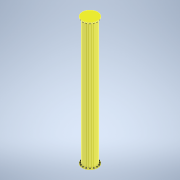
# Autodesk Inventor part: diam1m_len10m_x32gon_bolts
Saved by Autodesk Inventor 2022 (Build 260153000, 153)
## iProperties
Created: 2021-12-16
Part Number: diam1m_len10m_x32gon_bolts
Material: Steel
Document SubType Name: Modeling
Designer: jpc
Density: 7.85 g/cm^3
Appearance: Plate
Mass: 6.15675e+07 g
Surface Area: 349231 cm^2
Volume: 7.84299e+06 cm^3
Author: jpc
Autodesk Inventor part; units mm, degrees
ref_plane "YZ Plane" through (0, 0, 0) normal (1, 0, 0) x (0, 1, 0)
ref_plane "XZ Plane" through (0, 0, 0) normal (0, 1, 0) x (-1, 0, 0)
ref_plane "XY Plane" through (0, 0, 0) normal (0, 0, 1) x (1, 0, 0)
sketch "Sketch1" plane through (0, 0, 0) normal (0, 1, 0) x (-1, 0, 0)
  circle A0 centre (0, 0) radius 500 construction
  line L0 (497.5924, 49.0086) -> (497.5924, -49.0086)
  line L1 (497.5924, -49.0086) -> (478.4702, -145.1423)
  line L2 (478.4702, -145.1423) -> (440.9606, -235.6984)
  line L3 (440.9606, -235.6984) -> (386.5052, -317.1966)
  line L4 (386.5052, -317.1966) -> (317.1966, -386.5052)
  line L5 (317.1966, -386.5052) -> (235.6984, -440.9606)
  line L6 (235.6984, -440.9606) -> (145.1423, -478.4702)
  line L7 (145.1423, -478.4702) -> (49.0086, -497.5924)
  line L8 (49.0086, -497.5924) -> (-49.0086, -497.5924)
  line L9 (-49.0086, -497.5924) -> (-145.1423, -478.4702)
  line L10 (-145.1423, -478.4702) -> (-235.6984, -440.9606)
  line L11 (-235.6984, -440.9606) -> (-317.1966, -386.5052)
  line L12 (-317.1966, -386.5052) -> (-386.5052, -317.1966)
  line L13 (-386.5052, -317.1966) -> (-440.9606, -235.6984)
  line L14 (-440.9606, -235.6984) -> (-478.4702, -145.1423)
  line L15 (-478.4702, -145.1423) -> (-497.5924, -49.0086)
  line L16 (-497.5924, -49.0086) -> (-497.5924, 49.0086)
  line L17 (-497.5924, 49.0086) -> (-478.4702, 145.1423)
  line L18 (-478.4702, 145.1423) -> (-440.9606, 235.6984)
  line L19 (-440.9606, 235.6984) -> (-386.5052, 317.1966)
  line L20 (-386.5052, 317.1966) -> (-317.1966, 386.5052)
  line L21 (-317.1966, 386.5052) -> (-235.6984, 440.9606)
  line L22 (-235.6984, 440.9606) -> (-145.1423, 478.4702)
  line L23 (-145.1423, 478.4702) -> (-49.0086, 497.5924)
  line L24 (-49.0086, 497.5924) -> (49.0086, 497.5924)
  line L25 (49.0086, 497.5924) -> (145.1423, 478.4702)
  line L26 (145.1423, 478.4702) -> (235.6984, 440.9606)
  line L27 (235.6984, 440.9606) -> (317.1966, 386.5052)
  line L28 (317.1966, 386.5052) -> (386.5052, 317.1966)
  line L29 (386.5052, 317.1966) -> (440.9606, 235.6984)
  line L30 (440.9606, 235.6984) -> (478.4702, 145.1423)
  line L31 (478.4702, 145.1423) -> (497.5924, 49.0086)
  dimension "diamO" = 1000
  constraints: 64 end point, 2 coincident, 1 vertical, 68 other
extrude "Cylinder" add sketch "Sketch1" along normal blind 10000
sketch "Sketch2" plane through (0, 0, 0) normal (0, -1, 0) x (1, 0, 0)
  circle A0 centre (0, 0) radius 600 construction
  line L0 (597.1108, 58.8103) -> (597.1108, -58.8103)
  line L1 (597.1108, -58.8103) -> (574.1642, -174.1708)
  line L2 (574.1642, -174.1708) -> (529.1528, -282.838)
  line L3 (529.1528, -282.838) -> (463.8063, -380.636)
  line L4 (463.8063, -380.636) -> (380.636, -463.8063)
  line L5 (380.636, -463.8063) -> (282.838, -529.1528)
  line L6 (282.838, -529.1528) -> (174.1708, -574.1642)
  line L7 (174.1708, -574.1642) -> (58.8103, -597.1108)
  line L8 (58.8103, -597.1108) -> (-58.8103, -597.1108)
  line L9 (-58.8103, -597.1108) -> (-174.1708, -574.1642)
  line L10 (-174.1708, -574.1642) -> (-282.838, -529.1528)
  line L11 (-282.838, -529.1528) -> (-380.636, -463.8063)
  line L12 (-380.636, -463.8063) -> (-463.8063, -380.636)
  line L13 (-463.8063, -380.636) -> (-529.1528, -282.838)
  line L14 (-529.1528, -282.838) -> (-574.1642, -174.1708)
  line L15 (-574.1642, -174.1708) -> (-597.1108, -58.8103)
  line L16 (-597.1108, -58.8103) -> (-597.1108, 58.8103)
  line L17 (-597.1108, 58.8103) -> (-574.1642, 174.1708)
  line L18 (-574.1642, 174.1708) -> (-529.1528, 282.838)
  line L19 (-529.1528, 282.838) -> (-463.8063, 380.636)
  line L20 (-463.8063, 380.636) -> (-380.636, 463.8063)
  line L21 (-380.636, 463.8063) -> (-282.838, 529.1528)
  line L22 (-282.838, 529.1528) -> (-174.1708, 574.1642)
  line L23 (-174.1708, 574.1642) -> (-58.8103, 597.1108)
  line L24 (-58.8103, 597.1108) -> (58.8103, 597.1108)
  line L25 (58.8103, 597.1108) -> (174.1708, 574.1642)
  line L26 (174.1708, 574.1642) -> (282.838, 529.1528)
  line L27 (282.838, 529.1528) -> (380.636, 463.8063)
  line L28 (380.636, 463.8063) -> (463.8063, 380.636)
  line L29 (463.8063, 380.636) -> (529.1528, 282.838)
  line L30 (529.1528, 282.838) -> (574.1642, 174.1708)
  line L31 (574.1642, 174.1708) -> (597.1108, 58.8103)
  dimension "d3" = 1200
  constraints: 64 end point, 2 coincident, 1 vertical, 68 other
extrude "Endcap" add sketch "Sketch2" against normal blind 50
ref_plane "Midplane" through (0, 5000, 0) normal (0, 1, 0) x (1, 0, 0)
mirror "MirroredEndcap" about plane through (0, 5000, 0) normal (0, 1, 0) of "Endcap", "Cylinder"
sketch "Sketch3" plane through (0, 50, 0) normal (0, 1, 0) x (1, 0, 0)
  line L0 (529.1528, -282.838) -> (463.8063, -380.636) construction
  line L1 (463.8063, -380.636) -> (380.636, -463.8063) construction
  line L2 (380.636, -463.8063) -> (282.838, -529.1528) construction
  line L3 (282.838, -529.1528) -> (174.1708, -574.1642) construction
  line L4 (174.1708, -574.1642) -> (58.8103, -597.1108) construction
  line L5 (58.8103, -597.1108) -> (-58.8103, -597.1108) construction
  line L6 (-58.8103, -597.1108) -> (-174.1708, -574.1642) construction
  line L7 (-174.1708, -574.1642) -> (-282.838, -529.1528) construction
  line L8 (-282.838, -529.1528) -> (-380.636, -463.8063) construction
  line L9 (-380.636, -463.8063) -> (-463.8063, -380.636) construction
  line L10 (-463.8063, -380.636) -> (-529.1528, -282.838) construction
  line L11 (-529.1528, -282.838) -> (-574.1642, -174.1708) construction
  line L12 (-574.1642, -174.1708) -> (-597.1108, -58.8103) construction
  line L13 (-597.1108, -58.8103) -> (-597.1108, 58.8103) construction
  line L14 (-597.1108, 58.8103) -> (-574.1642, 174.1708) construction
  line L15 (-574.1642, 174.1708) -> (-529.1528, 282.838) construction
  line L16 (-529.1528, 282.838) -> (-463.8063, 380.636) construction
  line L17 (-463.8063, 380.636) -> (-380.636, 463.8063) construction
  line L18 (-380.636, 463.8063) -> (-282.838, 529.1528) construction
  line L19 (-282.838, 529.1528) -> (-174.1708, 574.1642) construction
  line L20 (-174.1708, 574.1642) -> (-58.8103, 597.1108) construction
  line L21 (-58.8103, 597.1108) -> (58.8103, 597.1108) construction
  line L22 (58.8103, 597.1108) -> (174.1708, 574.1642) construction
  line L23 (174.1708, 574.1642) -> (282.838, 529.1528) construction
  line L24 (282.838, 529.1528) -> (380.636, 463.8063) construction
  line L25 (380.636, 463.8063) -> (463.8063, 380.636) construction
  line L26 (463.8063, 380.636) -> (529.1528, 282.838) construction
  line L27 (529.1528, 282.838) -> (574.1642, 174.1708) construction
  line L28 (574.1642, 174.1708) -> (597.1108, 58.8103) construction
  line L29 (597.1108, 58.8103) -> (597.1108, -58.8103) construction
  line L30 (597.1108, -58.8103) -> (574.1642, -174.1708) construction
  line L31 (574.1642, -174.1708) -> (529.1528, -282.838) construction
  line L32 (478.4702, 145.1423) -> (497.5924, 49.0086) construction
  line L33 (497.5924, 49.0086) -> (497.5924, -49.0086) construction
  line L34 (497.5924, -49.0086) -> (478.4702, -145.1423) construction
  line L35 (478.4702, -145.1423) -> (440.9606, -235.6984) construction
  line L36 (440.9606, -235.6984) -> (386.5052, -317.1966) construction
  line L37 (386.5052, -317.1966) -> (317.1966, -386.5052) construction
  line L38 (317.1966, -386.5052) -> (235.6984, -440.9606) construction
  line L39 (235.6984, -440.9606) -> (145.1423, -478.4702) construction
  line L40 (145.1423, -478.4702) -> (49.0086, -497.5924) construction
  line L41 (49.0086, -497.5924) -> (-49.0086, -497.5924) construction
  line L42 (-49.0086, -497.5924) -> (-145.1423, -478.4702) construction
  line L43 (-145.1423, -478.4702) -> (-235.6984, -440.9606) construction
  line L44 (-235.6984, -440.9606) -> (-317.1966, -386.5052) construction
  line L45 (-317.1966, -386.5052) -> (-386.5052, -317.1966) construction
  line L46 (-386.5052, -317.1966) -> (-440.9606, -235.6984) construction
  line L47 (-440.9606, -235.6984) -> (-478.4702, -145.1423) construction
  line L48 (-478.4702, -145.1423) -> (-497.5924, -49.0086) construction
  line L49 (-497.5924, -49.0086) -> (-497.5924, 49.0086) construction
  line L50 (-497.5924, 49.0086) -> (-478.4702, 145.1423) construction
  line L51 (-478.4702, 145.1423) -> (-440.9606, 235.6984) construction
  line L52 (-440.9606, 235.6984) -> (-386.5052, 317.1966) construction
  line L53 (-386.5052, 317.1966) -> (-317.1966, 386.5052) construction
  line L54 (-317.1966, 386.5052) -> (-235.6984, 440.9606) construction
  line L55 (-235.6984, 440.9606) -> (-145.1423, 478.4702) construction
  line L56 (-145.1423, 478.4702) -> (-49.0086, 497.5924) construction
  line L57 (-49.0086, 497.5924) -> (49.0086, 497.5924) construction
  line L58 (49.0086, 497.5924) -> (145.1423, 478.4702) construction
  line L59 (145.1423, 478.4702) -> (235.6984, 440.9606) construction
  line L60 (235.6984, 440.9606) -> (317.1966, 386.5052) construction
  line L61 (317.1966, 386.5052) -> (386.5052, 317.1966) construction
  line L62 (386.5052, 317.1966) -> (440.9606, 235.6984) construction
  line L63 (440.9606, 235.6984) -> (478.4702, 145.1423) construction
  line L64 (-58.8103, 597.1108) -> (58.8103, 597.1108) construction
  line L65 (0, 597.1108) -> (0, 497.5924) construction
  circle A0 centre (0, 547.3516) radius 31.0995 construction
  line L66 (17.9553, 578.4511) -> (35.9106, 547.3516)
  line L67 (35.9106, 547.3516) -> (17.9553, 516.2521)
  line L68 (17.9553, 516.2521) -> (-17.9553, 516.2521)
  line L69 (-17.9553, 516.2521) -> (-35.9106, 547.3516)
  line L70 (-35.9106, 547.3516) -> (-17.9553, 578.4511)
  line L71 (-17.9553, 578.4511) -> (17.9553, 578.4511)
  point P0 (0, 0)
  point P1 (0, 578.4511)
  dimension "d7" = 62.199
  dimension "d6" = 99.5185
  constraints: 14 end point, 4 midpoint, 1 coincident, 1 point on line, 1 vertical alignment, 15 other
  measures "d6" distance of L65.start L65.end
extrude "BoltHead" add sketch "Sketch3" along normal blind 37.5 separate body
pattern_circular "BoltHeads" count 16 over 360 about axis through (0, -10, 0) along (0, 1, 0) bodies 2
mirror "MirroredBolts" about plane through (0, 5000, 0) normal (0, 1, 0) bodies 2
sketch "Sketch4" plane through (519.4293, 9912.5, 176.2853) normal (0, -1, 0) x (0.7933533, 0, -0.6087614)
  line L0 (-211.4706, 115.0937) -> (-197.7282, 81.9166) construction
  line L1 (-247.074, 119.781) -> (-211.4706, 115.0937) construction
  line L2 (-268.935, 91.2911) -> (-247.074, 119.781) construction
  line L3 (-255.1926, 58.114) -> (-268.935, 91.2911) construction
  line L4 (-219.5892, 53.4268) -> (-255.1926, 58.114) construction
  line L5 (-197.7282, 81.9166) -> (-219.5892, 53.4268) construction
  circle A0 centre (-233.3316, 86.6039) radius 31.0995 construction
  line L6 (-247.074, 119.781) -> (-211.4706, 115.0937) construction
  line L7 (-197.7282, 81.9166) -> (-219.5892, 53.4268) construction
  circle A1 centre (-233.3316, 86.6039) radius 23.3246 construction
  line L8 (-233.3316, 109.9285) -> (-228.7812, 109.4803)
  line L9 (-228.7812, 109.4803) -> (-224.4056, 108.153)
  line L10 (-224.4056, 108.153) -> (-220.3731, 105.9976)
  line L11 (-220.3731, 105.9976) -> (-216.8386, 103.0969)
  line L12 (-216.8386, 103.0969) -> (-213.9379, 99.5623)
  line L13 (-213.9379, 99.5623) -> (-211.7824, 95.5298)
  line L14 (-211.7824, 95.5298) -> (-210.4551, 91.1543)
  line L15 (-210.4551, 91.1543) -> (-210.007, 86.6039)
  line L16 (-210.007, 86.6039) -> (-210.4551, 82.0534)
  line L17 (-210.4551, 82.0534) -> (-211.7824, 77.6779)
  line L18 (-211.7824, 77.6779) -> (-213.9379, 73.6454)
  line L19 (-213.9379, 73.6454) -> (-216.8386, 70.1108)
  line L20 (-216.8386, 70.1108) -> (-220.3731, 67.2101)
  line L21 (-220.3731, 67.2101) -> (-224.4056, 65.0547)
  line L22 (-224.4056, 65.0547) -> (-228.7812, 63.7274)
  line L23 (-228.7812, 63.7274) -> (-233.3316, 63.2792)
  line L24 (-233.3316, 63.2792) -> (-237.882, 63.7274)
  line L25 (-237.882, 63.7274) -> (-242.2576, 65.0547)
  line L26 (-242.2576, 65.0547) -> (-246.2901, 67.2101)
  line L27 (-246.2901, 67.2101) -> (-249.8246, 70.1108)
  line L28 (-249.8246, 70.1108) -> (-252.7253, 73.6454)
  line L29 (-252.7253, 73.6454) -> (-254.8808, 77.6779)
  line L30 (-254.8808, 77.6779) -> (-256.2081, 82.0534)
  line L31 (-256.2081, 82.0534) -> (-256.6562, 86.6039)
  line L32 (-256.6562, 86.6039) -> (-256.2081, 91.1543)
  line L33 (-256.2081, 91.1543) -> (-254.8808, 95.5298)
  line L34 (-254.8808, 95.5298) -> (-252.7253, 99.5623)
  line L35 (-252.7253, 99.5623) -> (-249.8246, 103.0969)
  line L36 (-249.8246, 103.0969) -> (-246.2901, 105.9976)
  line L37 (-246.2901, 105.9976) -> (-242.2576, 108.153)
  line L38 (-242.2576, 108.153) -> (-237.882, 109.4803)
  line L39 (-237.882, 109.4803) -> (-233.3316, 109.9285)
  point P0 (-304.7753, -456.0651)
  dimension "d14" = 46.6493
  dimension "d13" = 62.199
  constraints: 64 end point, 3 tangent, 2 coincident, 1 centre point, 1 vertical alignment, 67 other
  measures "d13" diameter of A0
extrude "BoltThread" add sketch "Sketch4" along normal blind 37.5 bodies 2
pattern_circular "Circular Pattern2" count 16 over 360 about axis through (0, -10, 0) along (0, 1, 0) of "BoltThread" bodies 2
equation "\"d3\" = 1.2 * diamO"
equation "\"endcapThick\" = 0.005 * len"
equation "\"d7\" = 0.625 * d6"
equation "\"boltThick\" = 0.75 * endcapThick"
equation "\"d14\" = 0.75 * d13"
equation "\"d15\" = boltThick"
equation "\"len\" = 10000"
